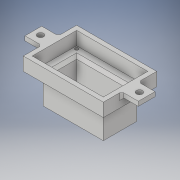
# Autodesk Inventor part: baza
Saved by Autodesk Inventor 2019 (Build 230136000, 136)
## iProperties
Created: 2019-08-06
Part Number: baza
Material: Ogólny
Document SubType Name: Modeling
Designer: mikol
Density: 1 g/cm^3
Appearance: Domyślna
Author: mikol
Autodesk Inventor part; units mm, degrees
ref_plane "YZ Plane" through (0, 0, 0) normal (1, 0, 0) x (0, 1, 0)
ref_plane "XZ Plane" through (0, 0, 0) normal (0, 1, 0) x (-1, 0, 0)
ref_plane "XY Plane" through (0, 0, 0) normal (0, 0, 1) x (1, 0, 0)
sketch "Szkic3" plane through (0, 0, 0) normal (0, 1, 0) x (-1, 0, 0)
  line L0 (27, 15) -> (-27, 15)
  line L1 (-27, 15) -> (-27, -15)
  line L2 (-27, -15) -> (27, -15)
  line L3 (27, -15) -> (27, 15)
  line L4 (27, 15) -> (-27, -15) construction
  line L5 (-27, 15) -> (27, -15) construction
  point P0 (0, 0)
  dimension "d2" = 54
  dimension "d3" = 30
  constraints: 12 end point, 2 midpoint, 2 parallel, 1 horizontal, 1 perpendicular
  measures "d2" distance of L2.end L1.end
  measures "d3" distance of L1.end L0.end
extrude "Wyciągnięcie proste1" add sketch "Szkic3" along normal blind 3
sketch "Szkic4" plane through (0, 3, 0) normal (0, 1, 0) x (1, 0, 0)
  circle A0 centre (-12.75, 0) radius 8.05
  circle A1 centre (12.75, 0) radius 8.05
  line L0 (27, 15) -> (-27, 15) projected
  line L1 (27, -15) -> (27, 15) projected
  line L2 (-27, 15) -> (-27, -15) projected
  line L3 (-27, -15) -> (27, -15) projected
  point P0 (0, 0)
  dimension "d6" = 16.1
  dimension "d7" = 16.1
  dimension "d8" = 25.5
  dimension "d9" = 15
  dimension "d10" = 15
  dimension "d11" = 14.25
  dimension "d12" = 14.25
  dimension "d15" = 15
  dimension "d16" = 15
  constraints: 2 centre point
  measures "d6" diameter of A0
  measures "d7" diameter of A1
  measures "d8" distance of A1.centre A0.centre
  measures "d9" distance from line of L0 A0.centre
  measures "d10" distance from line of L0 A1.centre
  measures "d11" distance from line of L1 A1.centre
  measures "d12" distance from line of L2 A0.centre
  measures "d15" distance from line of L3 A0.centre
  measures "d16" distance from line of L3 A1.centre
extrude "Wyciągnięcie proste2" cut sketch "Szkic4" against normal blind 3 contours A0 | A1
sketch "Szkic5" plane through (0, 3, 0) normal (0, 1, 0) x (1, 0, 0)
  circle A0 centre (-12.75, 0) radius 8.05 projected
  circle A1 centre (12.75, 0) radius 8.05 projected
  line L0 (-27, -15) -> (27, -15) projected
  line L1 (27, -15) -> (27, 15) projected
  line L2 (27, 15) -> (-27, 15) projected
  line L3 (-27, 15) -> (-27, -15) projected
  line L4 (-27, 15) -> (27, 15)
  line L5 (27, 15) -> (27, -15)
  line L6 (27, -15) -> (-27, -15)
  line L7 (-27, -15) -> (-27, 15)
  line L8 (-24, 12) -> (24, 12)
  line L9 (24, 12) -> (24, -12)
  line L10 (24, -12) -> (-24, -12)
  line L11 (-24, -12) -> (-24, 12)
  point P0 (0, 0)
  dimension "d17" = 3
  dimension "d18" = 3
  dimension "d19" = 3
  dimension "d20" = 3
  constraints: 16 end point, 4 parallel, 2 horizontal, 2 perpendicular
  measures "d17" distance between parallel lines of L2 L8
  measures "d18" distance between parallel lines of L3 L11
  measures "d19" distance between parallel lines of L10 L0
  measures "d20" distance between parallel lines of L1 L9
extrude "Wyciągnięcie proste3" add sketch "Szkic5" along normal blind 23 contours L3 L2 L1 L0
sketch "Szkic6" plane through (0, 26, 0) normal (0, 1, 0) x (1, 0, 0)
  line L0 (-32, -20) -> (32, -20)
  line L1 (32, -20) -> (32, 20)
  line L2 (32, 20) -> (-32, 20)
  line L3 (-32, 20) -> (-32, -20)
  line L4 (-32, -20) -> (32, 20) construction
  line L5 (32, -20) -> (-32, 20) construction
  line L6 (24, 12) -> (24, -12) projected
  line L7 (24, -12) -> (-24, -12) projected
  line L8 (-24, -12) -> (-24, 12) projected
  line L9 (-24, 12) -> (24, 12) projected
  line L10 (27, -15) -> (27, 15) projected
  line L11 (27, 15) -> (-27, 15) projected
  line L12 (-27, 15) -> (-27, -15) projected
  line L13 (-27, -15) -> (27, -15) projected
  line L14 (-24, -12) -> (24, -12)
  line L15 (24, -12) -> (24, 12)
  line L16 (24, 12) -> (-24, 12)
  line L17 (-24, 12) -> (-24, -12)
  line L18 (-24, -12) -> (24, 12) construction
  line L19 (24, -12) -> (-24, 12) construction
  point P0 (0, 0)
  dimension "d23" = 64
  dimension "d24" = 40
  constraints: 24 end point, 4 midpoint, 4 parallel, 2 horizontal, 2 perpendicular
  measures "d23" distance of L2.end L1.end
  measures "d24" distance of L2.end L0.start
extrude "Wyciągnięcie proste4" add sketch "Szkic6" along normal blind 3 contours L3 L2 L1 L0
sketch "Szkic7" plane through (0, 29, 0) normal (0, 1, 0) x (1, 0, 0)
  circle A0 centre (-29.5, -17.5) radius 1.5
  line L0 (27, -15) -> (-27, -15) projected
  line L1 (-27, -15) -> (-27, 15) projected
  line L2 (-27, 15) -> (27, 15) projected
  line L3 (27, 15) -> (27, -15) projected
  line L4 (-32, -20) -> (32, -20) projected
  line L5 (32, -20) -> (32, 20) projected
  line L6 (32, 20) -> (-32, 20) projected
  line L7 (-32, 20) -> (-32, -20) projected
  circle A1 centre (-29.5, 17.5) radius 1.5
  circle A2 centre (29.5, -17.5) radius 1.5
  circle A3 centre (29.5, 17.5) radius 1.5
  point P0 (0, 0)
  dimension "d27" = 3
  dimension "d30" = 35
  dimension "d33" = 59
  dimension "d36" = 2.5
  dimension "d37" = 2.5
  dimension "d38" = 2.5
  constraints: 4 centre point, 1 horizontal, 1 vertical, 6 other
  measures "d27" diameter of A0
  measures "d30" distance of A0.centre A1.centre
  measures "d33" distance of A0.centre A2.centre
  measures "d36" distance from line of L7 A1.centre
  measures "d37" distance from line of L5 A3.centre
  measures "d38" distance from line of L4 A2.centre
extrude "Wyciągnięcie proste5" cut sketch "Szkic7" against normal through all contours A0 | A1 | A2 | A3
sketch "Szkic8" plane through (0, 29, 0) normal (0, 1, 0) x (1, 0, 0)
  line L0 (-36, -24) -> (36, -24)
  line L1 (36, -24) -> (36, 24)
  line L2 (36, 24) -> (-36, 24)
  line L3 (-36, 24) -> (-36, -24)
  line L4 (-36, -24) -> (36, 24) construction
  line L5 (36, -24) -> (-36, 24) construction
  line L6 (32, -20) -> (32, 20) projected
  line L7 (-32, -20) -> (32, -20)
  line L8 (32, -20) -> (32, 20)
  line L9 (32, 20) -> (-32, 20)
  line L10 (-32, 20) -> (-32, -20)
  line L11 (-32, -20) -> (32, 20) construction
  line L12 (32, -20) -> (-32, 20) construction
  point P0 (0, 0)
  dimension "d41" = 72
  dimension "d42" = 48
  dimension "d43" = 64
  dimension "d44" = 40
  constraints: 24 end point, 4 midpoint, 4 parallel, 2 horizontal, 2 perpendicular
  measures "d41" distance of L2.end L1.end
  measures "d42" distance of L0.end L1.end
  measures "d43" distance of L9.end L6.end
  measures "d44" distance of L6.end L7.end
extrude "Wyciągnięcie proste6" add sketch "Szkic8" along normal blind 12
sketch "Szkic9" plane through (0, 26, 0) normal (0, 1, 0) x (1, 0, 0)
  line L0 (24, 12) -> (24, -12) projected
  line L1 (24, -12) -> (-24, -12) projected
  line L2 (-24, -12) -> (-24, 12) projected
  line L3 (-24, 12) -> (24, 12) projected
  line L4 (27, -15) -> (27, 15) projected
  line L5 (27, 15) -> (-27, 15) projected
  line L6 (-27, 15) -> (-27, -15) projected
  line L7 (-27, -15) -> (27, -15) projected
  circle A0 centre (29.5, -17.5) radius 1.5 projected
  circle A1 centre (-29.5, -17.5) radius 1.5 projected
  circle A2 centre (-29.5, 17.5) radius 1.5 projected
  circle A3 centre (29.5, 17.5) radius 1.5 projected
  line L8 (27, -15) -> (-27, -15) projected
  line L9 (-27, -15) -> (-27, 15) projected
  line L10 (-27, 15) -> (27, 15) projected
  line L11 (27, 15) -> (27, -15) projected
  line L12 (-32, -20) -> (32, -20) projected
  line L13 (32, -20) -> (32, 20) projected
  line L14 (32, 20) -> (-32, 20) projected
  line L15 (-32, 20) -> (-32, -20) projected
  line L16 (27, 15) -> (27, -15) projected
  line L17 (-27, 15) -> (27, 15)
  line L18 (27, 15) -> (27, -15)
  line L19 (27, -15) -> (-27, -15)
  line L20 (-27, -15) -> (-27, 15)
  line L21 (-27, 15) -> (27, -15) construction
  line L22 (27, 15) -> (-27, -15) construction
  line L23 (-24, 12) -> (24, 12)
  line L24 (24, 12) -> (24, -12)
  line L25 (24, -12) -> (-24, -12)
  line L26 (-24, -12) -> (-24, 12)
  line L27 (-24, 12) -> (24, -12) construction
  line L28 (24, 12) -> (-24, -12) construction
  point P0 (0, 0)
  constraints: 24 end point, 4 midpoint, 4 parallel, 2 horizontal, 2 perpendicular
extrude "Wyciągnięcie proste7" add sketch "Szkic9" along normal blind 3 contours L7 L6 L5 L4
chamfer "Faza1" distance 2.5 angle 45 4 edges at (0, 29, -12) (-24, 29, 0) (24, 29, 0) (0, 29, 12)
sketch "Szkic10" plane through (0, 29, 0) normal (0, -1, 0) x (1, 0, 0)
  line L0 (-32, -20) -> (-32, 20) projected
  line L1 (-32, 20) -> (32, 20) projected
  line L2 (32, 20) -> (32, -20) projected
  line L3 (32, -20) -> (-32, -20) projected
  line L4 (-36, 24) -> (36, 24) projected
  line L5 (-36, -24) -> (-36, 24) projected
  line L6 (36, -24) -> (-36, -24) projected
  line L7 (36, 24) -> (36, -24) projected
  line L8 (-32, -20) -> (32, -20)
  line L9 (32, -20) -> (32, 20)
  line L10 (32, 20) -> (-32, 20)
  line L11 (-32, 20) -> (-32, -20)
  line L12 (-32, -20) -> (32, 20) construction
  line L13 (32, -20) -> (-32, 20) construction
  line L14 (-36, -24) -> (36, -24)
  line L15 (36, -24) -> (36, 24)
  line L16 (36, 24) -> (-36, 24)
  line L17 (-36, 24) -> (-36, -24)
  line L18 (-36, -24) -> (36, 24) construction
  line L19 (36, -24) -> (-36, 24) construction
  point P0 (0, 0)
  constraints: 24 end point, 4 midpoint, 4 parallel, 2 horizontal, 2 perpendicular
extrude "Wyciągnięcie proste8" add sketch "Szkic10" along normal blind 3
chamfer "Faza2" distance 3 angle 45 4 edges at (0, 26, -24) (36, 26, 0) (0, 26, 24) (-36, 26, 0)
sketch "Szkic11" plane through (-36, 41, -24) normal (-1, 0, 0) x (0, 0, 1)
  line L0 (48, -12) -> (0, -12) projected
  line L1 (48, 0) -> (48, -12) projected
  line L2 (0, 0) -> (48, 0) projected
  line L3 (0, -12) -> (0, 0) projected
  line L4 (48, 0) -> (0, 0) projected
  line L5 (16.5, 0) -> (31.5, 0)
  line L6 (31.5, 0) -> (31.5, -4)
  line L7 (31.5, -4) -> (16.5, -4)
  line L8 (16.5, -4) -> (16.5, 0)
  point P0 (24, -41)
  dimension "d57" = 15
  dimension "d58" = 4
  dimension "d59" = 16.5
  dimension "d60" = 16.5
  constraints: 8 end point, 2 parallel, 1 horizontal, 1 perpendicular, 1 point on line
  measures "d57" distance of L6.end L7.end
  measures "d58" distance of L5.end L6.end
  measures "d59" distance between parallel lines of L1 L6
  measures "d60" distance between parallel lines of L3 L8
extrude "Wyciągnięcie proste9" add sketch "Szkic11" along normal blind 15 contours L6 L7 L8 L2
sketch "Szkic12" plane through (-36, 37, -7.5) normal (0, -1, 0) x (1, 0, 0)
  circle A0 centre (-8.5, 7.5) radius 2.75
  line L0 (0, 0) -> (-15, 0) projected
  line L1 (-15, 0) -> (-15, 15) projected
  point P0 (36, 7.5)
  dimension "d63" = 5.5
  dimension "d64" = 7.5
  dimension "d65" = 6.5
  constraints: 1 centre point
  measures "d63" diameter of A0
  measures "d64" distance from line of L0 A0.centre
  measures "d65" distance from line of L1 A0.centre
extrude "Wyciągnięcie proste10" cut sketch "Szkic12" against normal blind 15
mirror "Odbij1" about plane through (0, 0, 0) normal (1, 0, 0) of "Wyciągnięcie proste9", "Wyciągnięcie proste10"
chamfer "Faza3" distance 2 angle 45 1 edges at (36, 37, 0)
chamfer "Faza4" distance 2 angle 45 6 edges at (36, 36, 7.5) (36, 39, 7.5) (36, 36, -7.5) (36, 39, -7.5) (-36, 37, 0) (-36, 39, 7.5)
chamfer "Faza5" distance 2 angle 45 2 edges at (-36, 36, -7.5) (-36, 39, -7.5)
chamfer "Faza6" distance 2 angle 45 4 edges at (0, 0, 15) (-27, 0, 0) (0, 0, -15) (27, 0, 0)
equation "\"d9\" = d15"
equation "\"d10\" = d16"
equation "\"d11\" = d12"
equation "\"d36\" = d37"
equation "\"d59\" = d60"
